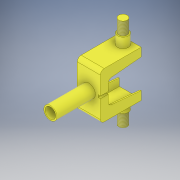
# Autodesk Inventor part: chassis
Saved by Autodesk Inventor 2017 (Build 210142000, 142)
## iProperties
Created: 2017-08-22
Part Number: chassis
Material: Generic
Document SubType Name: Modeling
Designer: MineV
Density: 1 g/cm^3
Appearance: Smooth - Yellow
Author: MineV
Autodesk Inventor part; units mm, degrees
ref_plane "YZ Plane" through (0, 0, 0) normal (1, 0, 0) x (0, 1, 0)
ref_plane "XZ Plane" through (0, 0, 0) normal (0, 1, 0) x (-1, 0, 0)
ref_plane "XY Plane" through (0, 0, 0) normal (0, 0, 1) x (1, 0, 0)
sketch "Sketch1" plane through (0, 0, 0) normal (1, 0, 0) x (0, 1, 0)
  line L0 (25, 4.96013) -> (-25, 4.96013)
  line L1 (-30, -0.03987) -> (-30, -48.03987)
  line L2 (-30, -48.03987) -> (30, -48.03987) construction
  line L3 (30, -48.03987) -> (30, -0.03987)
  line L4 (30, -48.03987) -> (19, -48.03987)
  line L5 (19, -48.03987) -> (15.422036, -9.576753)
  line L6 (10.44353, -5.03987) -> (-10.44353, -5.03987)
  line L7 (-15.422036, -9.576753) -> (-19, -48.03987)
  line L8 (-30, -48.03987) -> (-19, -48.03987)
  arc A0 (-25, 4.96013) -> (-30, -0.03987) centre (-25, -0.03987) ccw
  arc A1 (30, -0.03987) -> (25, 4.96013) centre (25, -0.03987) ccw
  arc A2 (-10.44353, -5.03987) -> (-15.422036, -9.576753) centre (-10.44353, -10.03987) ccw
  arc A3 (15.422036, -9.576753) -> (10.44353, -5.03987) centre (10.44353, -10.03987) ccw
  point P0 (0, 0)
  point P1 (30, 4.96013)
  point P2 (15, -5.03987)
  point P3 (-15, -5.03987)
  dimension "d0" = 60
  dimension "d1" = 53
  dimension "d2" = 10
  dimension "d3" = 11
  dimension "d4" = 11
  dimension "d5" = 30
  dimension "d6" = 15
  dimension "d7" = 30
  dimension "d8" = 5
  dimension "d11" = 5
  constraints: 18 end point, 8 point on circle, 8 point on line, 8 tangent, 4 centre point, 3 parallel, 2 equal radius, 1 collinear, 1 horizontal, 1 perpendicular
  measures "d0" distance of L1.end L2.end
  measures "d1" distance of L2.end point (30, 4.96)
  measures "d2" distance between parallel lines of L0 L6
  measures "d3" distance of L2.end L4.end
  measures "d4" distance of L1.end L7.end
  measures "d5" distance of point (15, -5.04) point (-15, -5.04)
  measures "d6" horizontal distance of point (0, 0) point (-15, -5.04)
  measures "d7" distance from line of point (0, 0) L1
  measures "d8" radius of A0
  measures "d11" radius of A2
extrude "Extrusion1" add sketch "Sketch1" along normal mid plane 30
sketch "Sketch2" plane through (-15, -25, 4.96013) normal (0, 0, 1) x (1, 0, 0)
  circle A0 centre (15, 25) radius 8.5
  dimension "d12" = 17
  constraints: 1 centre point, 1 coincident
  measures "d12" diameter of A0
extrude "Pin" add sketch "Sketch2" along normal blind 50
sketch "Sketch5" plane through (-15, -25, 4.96013) normal (0, 0, 1) x (1, 0, 0)
  line L0 (27, 26.5) -> (30, 26.5)
  line L1 (30, 26.5) -> (30, 23.5)
  line L2 (30, 23.5) -> (27, 23.5)
  line L3 (27, 23.5) -> (27, 26.5)
  line L4 (27, 26.5) -> (30, 23.5) construction
  line L5 (30, 26.5) -> (27, 23.5) construction
  line L6 (30, 50) -> (30, 0) projected
  point P0 (15, 25)
  point P1 (28.5, 25)
  dimension "d28" = 3
  dimension "d29" = 3
  dimension "d30" = 0
  constraints: 12 end point, 2 midpoint, 2 parallel, 1 horizontal, 1 perpendicular
  measures "d28" distance of L1.end L2.end
  measures "d29" distance of L0.end L1.end
  measures "d30" distance between parallel lines of L6 L1
extrude "Extrusion4" cut sketch "Sketch5" against normal through all
shell "Shell1" thickness 1.5875 removed faces 8 at (5, -26.333333, -48.03987) at (5, -15.367276, -9.169971) at (-6, -0.5, -5.03987) at (5, 15.006505, -7.995546) at (-5, 17.807345, -35.218831) at (5, -17.807345, -35.218831) at (-5, 26.333333, -48.03987) at (-2.12078, -1.878848, 54.96013)
sketch "Sketch3" plane through (0, 0, 0) normal (1, 0, 0) x (0, 1, 0)
  line L0 (-30, -48.03987) -> (-30, -0.03987)
  line L1 (-30, -32.414077) -> (-43, -32.414077)
  line L2 (-43, -32.414077) -> (-43, -33.914077)
  line L3 (-43, -33.914077) -> (-60, -33.914077)
  line L4 (-60, -33.914077) -> (-60, -39.414077)
  line L5 (-60, -39.414077) -> (-30, -39.414077)
  line L6 (-30, -32.414077) -> (-30, -39.414077)
  point P0 (0, 0)
  dimension "d16" = 13
  dimension "d17" = 17
  dimension "d18" = 1.5
  dimension "d19" = 5.5
  constraints: 12 end point, 3 perpendicular, 2 horizontal, 2 point on line, 1 collinear
  measures "d16" distance of L1.start L1.end
  measures "d17" distance of L2.end L3.end
  measures "d18" distance of L1.end L2.end
  measures "d19" distance of L3.end L4.end
revolve "Revolution1" add sketch "Sketch3" angle 360 about axis through (0, -60, -39.414077) along (0, 1, 0)
thread "Thread1" size "M11x1.5" class "6g" standard "ANSI Metric M Profile" full length
mirror "Mirror1" about plane through (0, 0, 0) normal (0, 1, 0) of "Revolution1"
equation "\"d4\" = d3"
equation "\"d6\" = 0.5 * d5"
equation "\"d7\" = 0.5 * d0"
body "Solid1"
